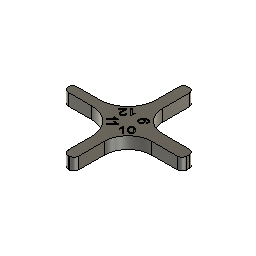
RadiusTool 9-12 v2 (Autodesk Fusion 360 design; units mm, degrees)
Autodesk Fusion 360 part; units mm, degrees
sketch "Sketch1" plane through (0, 0, 0) normal (0, 0, 1) x (1, 0, 0)
  circle A0 centre (0, 0) radius 25
  line L0 (-1.7886, 13.7886) -> (-1.7886, 24.9359)
  line L1 (-24.9359, 1.7886) -> (-13.7886, 1.7886)
  line L2 (24.887, -2.3744) -> (12.3744, -2.3744)
  line L3 (2.3744, -12.3744) -> (2.3744, -24.887)
  circle A1 centre (0, 0) radius 7.5 construction
  line L4 (0, 25) -> (0, -25) construction
  line L5 (2.6673, 11.6673) -> (2.6673, 24.8573)
  line L6 (11.6673, 2.6673) -> (24.8573, 2.6673)
  line L7 (-13.0815, -2.0815) -> (-24.9132, -2.0815)
  line L8 (-2.0815, -13.0815) -> (-2.0815, -24.9132)
  arc A2 (2.6673, 11.6673) -> (11.6673, 2.6673) centre (11.6673, 11.6673) ccw
  arc A3 (12.3744, -2.3744) -> (2.3744, -12.3744) centre (12.3744, -12.3744) ccw
  arc A4 (-2.0815, -13.0815) -> (-13.0815, -2.0815) centre (-13.0815, -13.0815) ccw
  arc A5 (-13.7886, 1.7886) -> (-1.7886, 13.7886) centre (-13.7886, 13.7886) ccw
  line L9 (-25, 0) -> (25, 0) construction
  dimension "d1" = 50
  dimension "d32" = 15
  dimension "d33" = 9
  dimension "d34" = 10
  dimension "d35" = 11
  dimension "d36" = 12
  constraint coincident A0.centre A1.centre
  constraint horizontal L2
  constraint vertical L3
  constraint horizontal L1
  constraint vertical L0
  constraint coincident A0 L4.start
  constraint coincident A0 L4.end
  constraint vertical L4
  constraint coincident A0.centre L4
  constraint coincident A0 L2.start
  constraint coincident A0 L3.end
  constraint coincident A0 L1.start
  constraint coincident A0 L0.end
  constraint coincident A0 L5.end
  constraint parallel L4 L5
  constraint coincident A0 L6.end
  constraint perpendicular L5 L6
  constraint coincident A0 L7.end
  constraint perpendicular L0 L7
  constraint coincident A0 L8.end
  constraint perpendicular L7 L8
  constraint tangent L5 A2
  constraint tangent L6 A2
  constraint tangent L3 A3
  constraint tangent L2 A3
  constraint tangent L7 A4
  constraint tangent L8 A4
  constraint tangent L1 A5
  constraint tangent L0 A5
  constraint tangent A1 A2
  constraint tangent A1 A3
  constraint tangent A1 A4
  constraint tangent A1 A5
  constraint coincident A0 L9.start
  constraint coincident A0 L9.end
  constraint parallel L2 L9
  constraint coincident A0.centre L9
  constraint equal L2 L3
  constraint equal L5 L6
  constraint equal L0 L1
  constraint equal L7 L8
  measures "d1" diameter of A0
  measures "d32" diameter of A1
  measures "d33" radius of A2
  measures "d34" radius of A3
  measures "d35" radius of A4
  measures "d36" radius of A5
extrude "Extrusion2" add sketch "Sketch1" along normal blind 5 contours A0 L0 L1 L2 L3 L5 L6 L7 L8 A2 A3 A4 A5
fillet "Abrundung1" radius 2 8 edges at (-24.9132, -2.0815, 2.5) (-24.9359, 1.7886, 2.5) (-1.7886, 24.9359, 2.5) (2.6673, 24.8573, 2.5) (24.8573, 2.6673, 2.5) (24.887, -2.3744, 2.5) (2.3744, -24.887, 2.5) (-2.0815, -24.9132, 2.5)
sketch "Skizze8" plane through (0, 0, 5) normal (0, 0, 1) x (-1, 0, 0)
  arc A0 (2.0815, 22.9999) -> (0.0886, 24.9998) centre (0.0815, 22.9999) ccw
  arc A1 (0.0886, 24.9998) -> (-0.4069, 24.9967) centre (0, 0) ccw
  arc A2 (-0.4069, 24.9967) -> (-2.3744, 22.997) centre (-0.3744, 22.997) ccw
  line L0 (-2.3744, 22.997) -> (-2.3744, 12.3744)
  arc A3 (-12.3744, 2.3744) -> (-2.3744, 12.3744) centre (-12.3744, 12.3744) ccw
  line L1 (-12.3744, 2.3744) -> (-22.997, 2.3744)
  arc A4 (-22.997, 2.3744) -> (-24.9967, 0.4069) centre (-22.997, 0.3744) ccw
  arc A5 (-24.9967, 0.4069) -> (-24.9895, -0.7253) centre (0, 0) ccw
  arc A6 (-24.9895, -0.7253) -> (-22.9903, -2.6673) centre (-22.9903, -0.6673) ccw
  line L2 (-22.9903, -2.6673) -> (-11.6673, -2.6673)
  arc A7 (-2.6673, -11.6673) -> (-11.6673, -2.6673) centre (-11.6673, -11.6673) ccw
  line L3 (-2.6673, -11.6673) -> (-2.6673, -22.9903)
  arc A8 (-2.6673, -22.9903) -> (-0.7253, -24.9895) centre (-0.6673, -22.9903) ccw
  arc A9 (-0.7253, -24.9895) -> (-0.2298, -24.9989) centre (0, 0) ccw
  arc A10 (-0.2298, -24.9989) -> (1.7886, -22.999) centre (-0.2114, -22.999) ccw
  line L4 (1.7886, -22.999) -> (1.7886, -13.7886)
  arc A11 (13.7886, -1.7886) -> (1.7886, -13.7886) centre (13.7886, -13.7886) ccw
  line L5 (13.7886, -1.7886) -> (23.0036, -1.7886)
  arc A12 (23.0036, -1.7886) -> (24.9998, 0.0886) centre (23.0036, 0.2114) ccw
  arc A13 (24.9998, 0.0886) -> (22.9999, 2.0815) centre (22.9999, 0.0815) ccw
  line L6 (22.9999, 2.0815) -> (13.0815, 2.0815)
  arc A14 (2.0815, 13.0815) -> (13.0815, 2.0815) centre (13.0815, 13.0815) ccw
  line L7 (2.0815, 13.0815) -> (2.0815, 22.9999)
  circle A15 centre (0, 0) radius 5.6053 construction
  line L8 (-5.3938, -3.7476) -> (-3.7296, -5.4118) construction
  line L9 (-3.7296, -5.4118) -> (-0.1941, -1.8763) construction
  line L10 (-0.1941, -1.8763) -> (-1.8583, -0.2121) construction
  line L11 (-1.8583, -0.2121) -> (-5.3938, -3.7476) construction
  line L12 (-2.6559, 6.3974) -> (-6.0343, 3.019) construction
  line L13 (-6.0343, 3.019) -> (-2.4988, -0.5166) construction
  line L14 (-2.4988, -0.5166) -> (0.8797, 2.8619) construction
  line L15 (0.8797, 2.8619) -> (-2.6559, 6.3974) construction
  line L16 (6.1379, 3.089) -> (3.5018, 5.7251) construction
  line L17 (3.5018, 5.7251) -> (-0.0338, 2.1896) construction
  line L18 (-0.0338, 2.1896) -> (2.6023, -0.4466) construction
  line L19 (2.6023, -0.4466) -> (6.1379, 3.089) construction
  line L20 (3.109, -6.0769) -> (6.4702, -2.7157) construction
  line L21 (6.4702, -2.7157) -> (2.9347, 0.8198) construction
  line L22 (2.9347, 0.8198) -> (-0.4265, -2.5413) construction
  line L23 (-0.4265, -2.5413) -> (3.109, -6.0769) construction
  text T0 "9" font "Arial" height 5 align ink ink in box 0 x 0 at (-5.3938, -3.7476) x (0.707107, -0.707107) y (0.707107, 0.707107) spacing 1 kerned height is em
  text T1 "10" font "Arial" height 5 align ink ink in box 0 x 0 at (-2.6559, 6.3974) x (-0.707107, -0.707107) y (0.707107, -0.707107) spacing 1 kerned height is em
  text T2 "11" font "Arial" height 5 align ink ink in box 0 x 0 at (6.1379, 3.089) x (-0.707107, 0.707107) y (-0.707107, -0.707107) spacing 1 kerned height is em
  text T3 "12" font "Arial" height 5 align ink ink in box 0 x 0 at (3.109, -6.0769) x (0.707107, 0.707107) y (-0.707107, 0.707107) spacing 1 kerned height is em
  constraint concentric A1 A15
  constraint perpendicular L8 L9
  constraint parallel L8 L10
  constraint parallel L9 L11
  constraint perpendicular L12 L13
  constraint parallel L12 L14
  constraint parallel L13 L15
  constraint perpendicular L16 L17
  constraint parallel L16 L18
  constraint parallel L17 L19
  constraint perpendicular L20 L21
  constraint parallel L20 L22
  constraint parallel L21 L23
extrude "Extrusion3" cut sketch "Skizze8" against normal blind 0.5 text T0 T1 T2 T3
